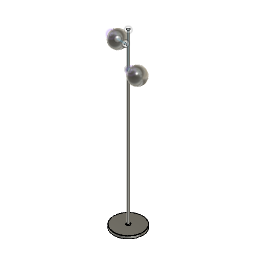
Week 4 HW Part 2 (Autodesk Fusion 360 design; units mm, degrees)
Autodesk Fusion 360 part; units mm, degrees
sketch "Sketch1" plane through (0, 0, 0) normal (0, 0, 1) x (1, 0, 0) in component "Base"
  circle A0 centre (0, 0) radius 139.7
  dimension "d1" = 279.4
  constraint coincident A0.centre origin
  measures "d1" diameter of A0
extrude "Extrude1" add sketch "Sketch1" along normal blind 25.4 makes body 1 in component "Base"
sketch "Sketch1 (2)" plane through (0, 0, 25.4) normal (0, 0, 1) x (-1, 0, 0) in component "Base connector"
  circle A0 centre (0, 0) radius 139.7
  circle A1 centre (0, 0) radius 19.05
  dimension "d4" = 38.1
  constraint concentric A0 A1
  measures "d4" diameter of A1
extrude "Extrude1'" add sketch "Sketch1 (2)" along normal blind 6.35 separate body contours A1 makes body 2 in component "Base connector"
chamfer "Chamfer1" distance 5.08 angle 35 1 edges at (17.7608, 6.8888, 31.75) measured on face at (-2.3199, 0.4007, 31.75) on bodies 2 in component "Base connector"
fillet "Fillet1" radius 2.54 1 edges at (-130.2461, -50.5177, 25.4) on bodies 1 in component "Base"
sketch "Sketch1 (3)" plane through (0, 0, 31.75) normal (0, 0, 1) x (-1, 0, 0) in component "Pole"
  circle A0 centre (0, 0) radius 13.97
  circle A1 centre (0, 0) radius 12.7
  dimension "d12" = 25.4
  constraint concentric A0 A1
  measures "d12" diameter of A1
extrude "Extrude1''" add sketch "Sketch1 (3)" along normal blind 1625.6 separate body contours A1 makes body 3 in component "Pole"
sketch "Sketch2" plane through (0, 0, 0) normal (1, 0, 0) x (0, 1, 0) in component "Pole"
  line L0 (0, 1651) -> (0, 1524)
  line L1 (0, 1524) -> (0, 1320.8)
  circle A0 centre (0, 1320.8) radius 10.16
  dimension "d15" = 127
  dimension "d20" = 203.2
  dimension "d21" = 20.32
  constraint vertical L0
  constraint parallel L0 L1
  constraint coincident L1.end A0.centre
  measures "d15" distance of L0.start L0.end
  measures "d20" distance of L0.end L1.end
  measures "d21" diameter of A0
hole "Hole1" at (0, 0, 1524) direction (-1, 0, 0) diameter 20.32 depth 25.4 tip angle 118 bodies 3 in component "Pole"
extrude "Extrude2" add sketch "Sketch2" along normal blind 25.4 bodies 3 in component "Pole"
sketch "Sketch1 (4)" plane through (25.4, 8.7057, 0.8935) normal (1, 0, 0) x (0, 1, 0) in component "Sphere"
  circle A0 centre (-8.7057, 1319.9065) radius 10.16
sketch "Sketch2 (2)" plane through (25.4, 0, 0) normal (1, 0, 0) x (0, 1, 0) in component "Sphere"
sphere "SpherePrimitive1" add diameter 152.4 placed x (1, 0, 0) y (0, 0, -1) z (0, 1, 0) at (97.033, -8.7057, 1320.0971) separate body makes body 4 in component "Sphere"
extrude "Extrude3" add 1 faces at (0, 0.0754, 1525.0067) along direction (-1, 0, 0) blind 25.4 on bodies 3 bodies 3 in component "Pole"
sketch "Sketch3" plane through (0, 0, 0) normal (0, 1, 0) x (1, 0, 0) in component "Pole"
  line L0 (-25.4, -1524) -> (-101.6, -1524)
  dimension "d29" = 76.2
  constraint horizontal L0
  measures "d29" distance of L0.start L0.end
sketch "Sketch2 (3)" plane through (0, 0, 0) normal (0, 1, 0) x (1, 0, 0)
copy_body "CopyPasteBodies1" bodies 4 makes body 5 in component "Sphere"
move_body "Move1" bodies 5 to x (1, 0, 0) y (0, 1, 0) z (0, 0, 1) at (0, 0, 0) in component "Sphere"
sketch "Sketch6" plane through (0, 0, 0) normal (0, 1, 0) x (1, 0, 0) in component "Sphere"
component "Base" placed x (1, 0, 0) y (0, 1, 0) z (0, 0, 1) at (0, 0, 0)
component "Base connector" placed x (1, 0, 0) y (0, 1, 0) z (0, 0, 1) at (0, 0, 0)
component "Pole" placed x (1, 0, 0) y (0, 1, 0) z (0, 0, 1) at (0, 0, 0)
component "Sphere" placed x (1, 0, 0) y (0, 1, 0) z (0, 0, 1) at (0, 0, 0)
component "Sphere" placed x (1, 0, 0) y (0, 1, 0) z (0, 0, 1) at (-198.633, 8.7057, 203.9029)
component "Component" placed x (1, 0, 0) y (0, 1, 0) z (0, 0, 1) at (0, 0, 0) in component "Base"
equation "d13 = ( 5 * 12 ) * 1 in + 4 in"
named bodies: "Light", "Holder"
